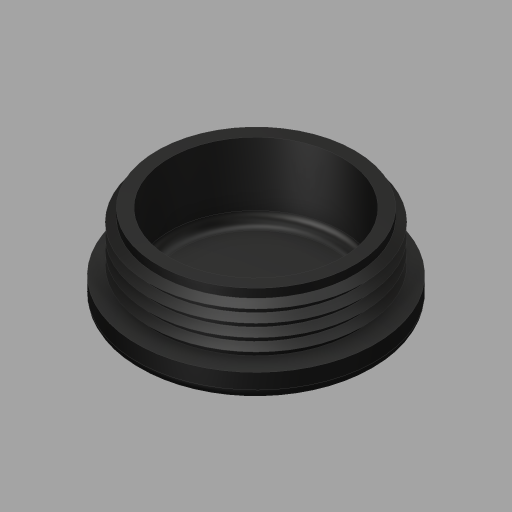
# Autodesk Inventor part: Round_sliders
Saved by Autodesk Inventor 2023.2 (Build 272271000, 271)
## iProperties
Created: 2023-02-02
Part Number: Round_sliders
Material: Generisch
Document SubType Name: Modeling
Designer: Raoul Messerli
Density: 1 g/cm^3
Appearance: Vorgabe
Author: Raoul Messerli
Autodesk Inventor part; units mm, degrees
ref_plane "YZ Plane" through (0, 0, 0) normal (1, 0, 0) x (0, 1, 0)
ref_plane "XZ Plane" through (0, 0, 0) normal (0, 1, 0) x (-1, 0, 0)
ref_plane "XY Plane" through (0, 0, 0) normal (0, 0, 1) x (1, 0, 0)
sketch "Skizze1" plane through (0, 0, 0) normal (1, 0, 0) x (0, 1, 0)
  line L0 (0, 0) -> (0, -24.7544)
  line L1 (17, 0) -> (21, 0)
  line L2 (21, 0) -> (21, -11.5)
  line L3 (21, -11.5) -> (23.5, -11.5)
  line L4 (23.5, -11.5) -> (23.5, -14.5)
  line L5 (21.5, -16.5) -> (0, -16.5)
  line L6 (17, 0) -> (17, -12.5)
  line L7 (15, -14.5) -> (0, -14.5)
  arc A0 (15, -14.5) -> (17, -12.5) centre (15, -12.5) ccw
  arc A1 (21.5, -16.5) -> (23.5, -14.5) centre (21.5, -14.5) ccw
  point P0 (23.5, -16.5)
  point P1 (21, -5.75)
  dimension "d0" = 42
  dimension "d1" = 47
  dimension "d2" = 5
  dimension "d3" = 11.5
  dimension "d5" = 2
  dimension "d6" = 2
  dimension "d8" = 4
  dimension "d9" = 2
  constraints: 16 end point, 5 point on line, 4 perpendicular, 4 point on circle, 4 tangent, 3 vertical, 2 centre point, 1 horizontal, 1 midpoint
  measures "d0" diameter of point (21, -5.75) L0
  measures "d1" diameter of L4 L0
  measures "d2" distance of L3.end point (23.5, -16.5)
  measures "d3" distance of L1.end L2.end
  measures "d5" radius of A0
  measures "d6" radius of A1
  measures "d8" distance between parallel lines of L6 L2
  measures "d9" distance between parallel lines of L5 L7
revolve "Umdrehung1" add sketch "Skizze1" angle 360 about axis through (0, 0, 0) along (0, 0, -1)
sketch "Skizze2" plane through (0, 0, 0) normal (1, 0, 0) x (0, 1, 0)
  line L0 (21, 0) -> (21, -11.5) projected
  line L1 (21, -11.5) -> (19.461, -11.5)
  line L2 (-23.5, -11.5) -> (23.5, -11.5) projected
  line L3 (19.461, -11.5) -> (19.461, -9.7922)
  line L4 (19.461, -9.7922) -> (21, -9.7922)
  line L5 (21, -9.7922) -> (19.461, -9.0519)
  line L6 (19.461, -9.0519) -> (19.461, -7.3442)
  line L7 (19.461, -7.3442) -> (21, -7.3442)
  line L8 (21, -7.3442) -> (19.461, -6.6039)
  line L9 (19.461, -6.6039) -> (19.461, -4.8961)
  line L10 (19.461, -4.8961) -> (21, -4.8961)
  line L11 (21, -4.8961) -> (19.461, -4.1558)
  line L12 (19.461, -4.1558) -> (19.461, -2.4481)
  line L13 (19.461, -2.4481) -> (21, -2.4481)
  line L14 (21, -2.4481) -> (19.461, -1.7078)
  line L15 (19.461, -1.7078) -> (19.461, 0)
  line L16 (-21, 0) -> (21, 0) projected
  line L17 (21, -11.5) -> (21, 0)
  line L18 (19.461, 0) -> (21, 0)
  line L19 (0, -19.8) -> (0, 3.3) projected
  point P0 (0, 0)
  constraints: 32 end point, 12 point on line, 8 equal length, 6 perpendicular, 3 parallel, 1 vertical
revolve "Umdrehung2" cut sketch "Skizze2" angle 360 about axis through (0, 0, -10) along (0, 0, 1) contours L0 L14 L15 L16 | L0 L11 L12 L13 | L0 L8 L9 L10 | L0 L5 L6 L7 | L0 L1 L3 L4
